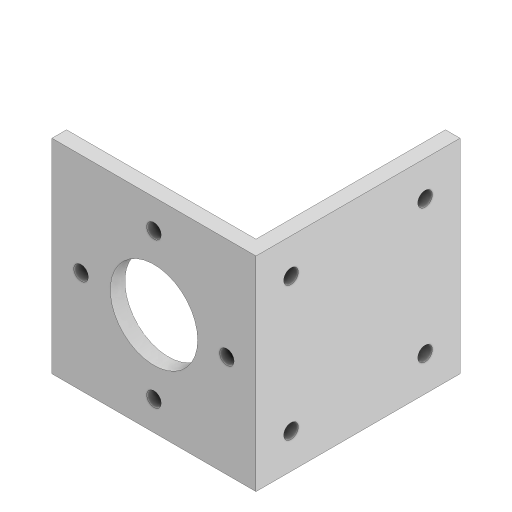
# Autodesk Inventor part: SOPORTE DE MOTOR
Saved by Autodesk Inventor 2024 (Build 280153000, 153)
## iProperties
Created: 2024-05-26
Part Number: SOPORTE DE MOTOR
Material: Generic
Document SubType Name: Modeling
Designer: Jhuliams
Density: 1 g/cm^3
Appearance: Default
Author: Jhuliams
Autodesk Inventor part; units mm, degrees
ref_plane "YZ Plane" through (0, 0, 0) normal (1, 0, 0) x (0, 1, 0)
ref_plane "XZ Plane" through (0, 0, 0) normal (0, 1, 0) x (-1, 0, 0)
ref_plane "XY Plane" through (0, 0, 0) normal (0, 0, 1) x (1, 0, 0)
sketch "Sketch1" plane through (0, 0, 0) normal (0, 0, 1) x (1, 0, 0)
  line L0 (-35, 35) -> (35, 35)
  line L1 (35, 35) -> (35, -35)
  line L2 (35, -35) -> (-35, -35)
  line L3 (-35, -35) -> (-35, 35)
  line L4 (-35, 35) -> (35, -35) construction
  line L5 (35, 35) -> (-35, -35) construction
  circle A0 centre (0, 0) radius 15
  circle A1 centre (0, 0) radius 25
  circle A2 centre (-25, 0) radius 2.5
  circle A3 centre (0, -25) radius 2.5
  circle A4 centre (25, 0) radius 2.5
  circle A5 centre (0, 25) radius 2.5
  dimension "d3" = 50
  dimension "d0" = 70
  dimension "d1" = 70
  dimension "d2" = 30
  dimension "d4" = 5
  dimension "d7" = 360
  constraints: 12 end point, 5 centre point, 2 coincident, 2 midpoint, 2 parallel, 1 horizontal, 1 horizontal alignment, 1 perpendicular, 11 other
  measures "d0" distance of L1.end L2.end
  measures "d1" distance of L0.end L1.end
  measures "d2" diameter of A0
  measures "d4" diameter of A2
extrude "Extrusion1" add sketch "Sketch1" along normal blind 5 contours L0 L1 L2 L3 | A4 A1 A3 A2 A5
sketch "Sketch2" plane through (35, -35, 0) normal (1, 0, 0) x (0, 0, -1)
  line L0 (-5, 0) -> (-5, 70) projected
  line L1 (-5, 70) -> (65, 70)
  line L2 (65, 70) -> (65, 0)
  line L3 (65, 0) -> (-5, 0)
  line L4 (-5, 0) -> (-5, 70)
  point P0 (0, 35)
  dimension "d11" = 70
  dimension "d12" = 70
  constraints: 8 end point, 2 parallel, 1 horizontal, 1 perpendicular
  measures "d11" distance of L2.end L3.end
  measures "d12" distance of L1.end L2.end
extrude "Extrusion2" add sketch "Sketch2" against normal blind 5
sketch "Sketch3" plane through (35, -35, 5) normal (1, 0, 0) x (0, 0, -1)
  line L0 (70, 70) -> (0, 70) projected
  line L1 (0, 0) -> (0, 70) projected
  line L2 (70, 0) -> (0, 0) projected
  line L3 (70, 0) -> (70, 70) projected
  line L4 (12, 58) -> (58, 58)
  line L5 (58, 58) -> (58, 12)
  line L6 (58, 12) -> (12, 12)
  line L7 (12, 12) -> (12, 58)
  circle A0 centre (12, 58) radius 2.5
  circle A1 centre (58, 58) radius 2.5
  circle A2 centre (12, 12) radius 2.5
  circle A3 centre (58, 12) radius 2.5
  point P0 (5, 35)
  dimension "d15" = 12
  dimension "d16" = 5
  dimension "d19" = 46
  dimension "d22" = 46
  constraints: 8 end point, 4 centre point, 1 coincident, 1 horizontal, 1 vertical, 9 other
  measures "d15" distance between parallel lines of L0 L4
  measures "d16" diameter of A0
  measures "d19" distance of A0.centre A1.centre
  measures "d22" distance of A0.centre A2.centre
extrude "Extrusion3" cut sketch "Sketch3" against normal blind 5 contours L7 A0 L4 | L4 A0 L7 | A1 L5 L4 | L4 L5 A1 | A2 L6 L7 | L7 L6 A2 | A3 L6 L5 | L5 L6 A3
body "Solid1"
